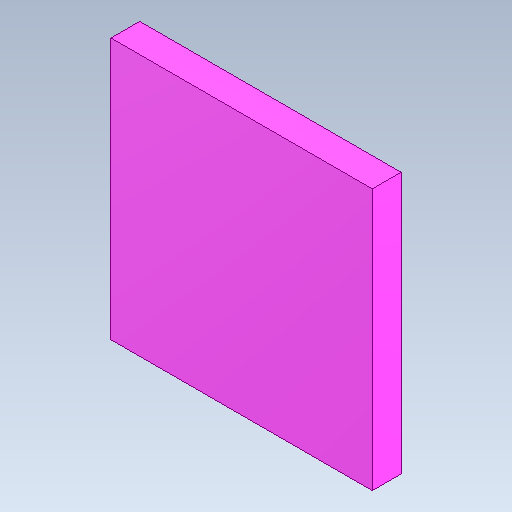
# Autodesk Inventor part: ATMEGA328
Saved by Autodesk Inventor 2020 (Build 240168000, 168)
## iProperties
Created: 2019-05-24
Part Number: ATMEGA328
Material: Generic
Document SubType Name: Modeling
Designer: psrob
Density: 1 g/cm^3
Appearance: TQFP32-08, ATMEGA328
Author: psrob
Autodesk Inventor part; units mm, degrees
ref_plane "YZ Plane" through (0, 0, 0) normal (1, 0, 0) x (0, 1, 0)
ref_plane "XZ Plane" through (0, 0, 0) normal (0, 1, 0) x (-1, 0, 0)
ref_plane "XY Plane" through (0, 0, 0) normal (0, 0, 1) x (1, 0, 0)
sketch "TQFP32-08, ATMEGA328_58" plane through (0, 0, 0) normal (0, 0, 1) x (1, 0, 0)
  line L0 (-4.5466, 4.5466) -> (4.5466, 4.5466)
  line L1 (4.5466, 4.5466) -> (4.5466, -4.5466)
  line L2 (4.5466, -4.5466) -> (-4.5466, -4.5466)
  line L3 (-4.5466, -4.5466) -> (-4.5466, 4.5466)
  constraints: 8 end point
extrude "Extrusion1" add sketch "TQFP32-08, ATMEGA328_58" along normal blind 1
body "Solid1"
